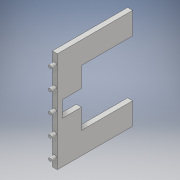
# Autodesk Inventor part: Back Plate V3
Saved by Autodesk Inventor 2017.3 (Build 213256000, 256)
## iProperties
Created: 2018-03-06
Part Number: Back Plate V3
Material: Generic
Document SubType Name: Modeling
Designer: Harsh Gupta
Density: 1 g/cm^3
Appearance: Default
Author: Harsh Gupta
Autodesk Inventor part; units mm, degrees
ref_plane "YZ Plane" through (0, 0, 0) normal (1, 0, 0) x (0, 1, 0)
ref_plane "XZ Plane" through (0, 0, 0) normal (0, 1, 0) x (-1, 0, 0)
sketch "Sketch2" plane through (0, 0, 0) normal (0, 1, 0) x (-1, 0, 0)
  line L0 (0, 0) -> (5, 0)
  line L1 (5, 0) -> (5, -100)
  line L2 (5, -100) -> (0, -100)
  line L3 (0, -100) -> (0, 0)
  dimension "d0" = 5
  dimension "d1" = 100
  constraints: 8 end point, 2 parallel, 1 horizontal, 1 perpendicular
  measures "d0" distance of L1.end L2.end
  measures "d1" distance of L0.end L1.end
extrude "Extrusion1" add sketch "Sketch2" along normal blind 75
sketch "Sketch5" plane through (0, 0, 0) normal (1, 0, 0) x (0, 0, -1)
  line L0 (0, 75) -> (100, 75) projected
  line L1 (22, 23.95) -> (42, 23.95)
  line L2 (42, 23.95) -> (42, 75)
  line L3 (42, 75) -> (22, 75)
  line L4 (22, 75) -> (22, 23.95)
  line L5 (58, 23.95) -> (78, 23.95)
  line L6 (78, 23.95) -> (78, 75)
  line L7 (78, 75) -> (58, 75)
  line L8 (58, 75) -> (58, 23.95)
  line L9 (0, 0) -> (0, 75) projected
  line L10 (100, 0) -> (100, 75) projected
  line L11 (100, 0) -> (0, 0) projected
  dimension "d16" = 16
  dimension "d17" = 22
  dimension "d18" = 22
  dimension "d20" = 23.95
  constraints: 16 end point, 4 parallel, 3 point on line, 2 horizontal, 2 perpendicular, 1 collinear
  measures "d16" distance between parallel lines of L8 L2
  measures "d17" distance between parallel lines of L4 L9
  measures "d18" distance between parallel lines of L10 L6
  measures "d20" distance between parallel lines of L11 L1
extrude "Extrusion4" cut sketch "Sketch5" against normal through all contours L0 L2 L1 L4 | L0 L6 L5 L8
sketch "Sketch6" plane through (0, 0, 0) normal (1, 0, 0) x (0, 0, -1)
  line L0 (58, 23.95) -> (58, 75) projected
  line L1 (42, 5) -> (58, 5)
  line L2 (58, 5) -> (58, 75)
  line L3 (58, 75) -> (42, 75)
  line L4 (42, 75) -> (42, 5)
  line L5 (42, 75) -> (42, 23.95) projected
  point P0 (0, 0)
  dimension "d26" = 70
  constraints: 8 end point, 2 parallel, 1 collinear, 1 horizontal, 1 perpendicular
  measures "d26" distance of L3.end L1.start
extrude "Extrusion5" cut sketch "Sketch6" against normal through all
sketch "Sketch7" plane through (0, 0, 0) normal (0, -1, 0) x (1, 0, 0)
  circle A0 centre (-2.5, -10) radius 1.5
  line L0 (0, 0) -> (-5, 0) projected
  line L1 (-5, 0) -> (-5, -100) projected
  dimension "d27" = 3
  dimension "d28" = 10
  dimension "d29" = 2.5
  constraints: 1 centre point
  measures "d27" diameter of A0
  measures "d28" distance from line of L0 A0.centre
  measures "d29" distance from line of L1 A0.centre
extrude "Extrusion6" add sketch "Sketch7" along normal blind 5
pattern_linear "Rectangular Pattern1" count 5 spacing 20 along (0, 0, -1) of "Extrusion6"
ref_plane "Work Plane1" through (-5, 0, -50) normal (0, 0, 1) x (1, 0, 0)
sketch "Sketch9" plane through (-5, -6.2824, -100) normal (-1, 0, 0) x (0, 0, 1)
  line L0 (100, 6.2824) -> (100, 75)
  line L1 (0, 29.2824) -> (100, 29.2824)
  line L2 (100, 29.2824) -> (100, 34.2824)
  line L3 (100, 34.2824) -> (0, 34.2824)
  line L4 (0, 34.2824) -> (0, 29.2824)
  circle A0 centre (92.5, 31.7824) radius 1.5
  line L5 (78, 75) -> (78, 23.95)
  line L6 (100, 75) -> (78, 75)
  line L7 (100, 6.2824) -> (95, 6.2824)
  line L8 (95, 6.2824) -> (95, 75)
  line L9 (95, 75) -> (100, 75)
  line L10 (100, 75) -> (100, 6.2824)
  line L11 (0, 75) -> (22, 75)
  line L12 (0, 0) -> (5, 0)
  line L13 (5, 0) -> (5, 75)
  line L14 (5, 75) -> (0, 75)
  line L15 (0, 75) -> (0, 0)
  point P0 (97.5, 6.2824)
  point P1 (100, 6.2824)
  dimension "d59" = 5
  dimension "d56" = 3
  dimension "d55" = 5
  dimension "d53" = 5
  dimension "d57" = 2.5
  dimension "d54" = 2.5
  dimension "d66" = 23
  constraints: 32 end point, 6 parallel, 3 horizontal, 3 perpendicular, 3 point on line, 1 centre point, 1 horizontal alignment, 1 midpoint
  measures "d59" distance of L2.end L1.end
  measures "d56" diameter of A0
  measures "d55" distance of L8.end L9.end
  measures "d53" distance of L14.end L13.end
  measures "d57" distance from line of L3 A0.centre
  measures "d54" distance from line of L8 A0.centre
  measures "d66" distance between parallel lines of L7 L1
extrude "Extrusion8" cut sketch "Sketch9" against normal blind 2.5 contours A0
pattern_linear "Rectangular Pattern3" count 3 spacing 6 along (0, 0, -1) of "Extrusion8"
mirror "Mirror2" about plane through (-5, 0, -50) normal (0, 0, 1) of "Extrusion8", "Rectangular Pattern3"
sketch "Sketch10" plane through (-5, 0, -100) normal (-1, 0, 0) x (0, 0, 1)
  line L0 (78, 75) -> (100, 75) projected
  line L1 (100, 0) -> (95, 0)
  line L2 (95, 0) -> (95, 75)
  line L3 (95, 75) -> (100, 75)
  line L4 (100, 75) -> (100, 0)
  circle A0 centre (97.5, 7.5) radius 1.5
  dimension "d67" = 5
  dimension "d68" = 3
  dimension "d69" = 2.5
  dimension "d70" = 7.5
  constraints: 8 end point, 2 parallel, 1 centre point, 1 horizontal, 1 perpendicular, 1 point on line
  measures "d67" distance of L2.end L3.end
  measures "d68" diameter of A0
  measures "d69" distance from line of L4 A0.centre
  measures "d70" distance from line of L1 A0.centre
extrude "Extrusion9" cut sketch "Sketch10" against normal blind 2.5 contours A0
pattern_linear "Rectangular Pattern4" count 3 spacing 30 along (0, 1, 0) of "Extrusion9"
mirror "Mirror3" about plane through (-5, 0, -50) normal (0, 0, 1) of "Extrusion9", "Rectangular Pattern4"
body "Solid1"
